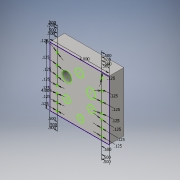
# Autodesk Inventor part: PopQuiz
Saved by Autodesk Inventor 2016 (Build 200138000, 138)
## iProperties
Created: 2018-02-16
Part Number: PopQuiz
Material: Generic
Document SubType Name: Modeling
Designer: sun01147
Density: 1 g/cm^3
Appearance: Default
Author: sun01147
Autodesk Inventor part; units mm, degrees
ref_plane "YZ Plane" through (0, 0, 0) normal (1, 0, 0) x (0, 1, 0)
ref_plane "XZ Plane" through (0, 0, 0) normal (0, 1, 0) x (-1, 0, 0)
ref_plane "XY Plane" through (0, 0, 0) normal (0, 0, 1) x (1, 0, 0)
sketch "Sketch1" plane through (0, 0, 0) normal (0, 0, 1) x (1, 0, 0)
  line L0 (0, 0) -> (0, 101.6)
  line L1 (0, 101.6) -> (101.6, 101.6)
  line L2 (101.6, 101.6) -> (101.6, 0)
  line L3 (101.6, 0) -> (0, 0)
  circle A0 centre (12.7, 92.4868) radius 1.5875
  circle A1 centre (12.7, 73.555) radius 1.5875
  circle A2 centre (12.7, 57.3937) radius 1.5875
  circle A3 centre (12.7, 43.772) radius 1.5875
  circle A4 centre (12.7, 31.3047) radius 1.5875
  circle A5 centre (12.7, 18.1448) radius 1.5875
  circle A6 centre (12.7, 5.9084) radius 1.5875
  circle A7 centre (88.9, 92.4868) radius 1.5875
  circle A8 centre (88.9, 73.555) radius 1.5875
  circle A9 centre (88.9, 57.3937) radius 1.5875
  circle A10 centre (88.9, 39.5628) radius 1.5875
  circle A11 centre (88.9, 31.3047) radius 1.5875
  circle A12 centre (88.9, 18.1448) radius 1.5875
  circle A13 centre (88.9, 5.9084) radius 1.5875
  circle A14 centre (50.8, 81.1516) radius 6.818
  circle A15 centre (29.171, 64.7351) radius 8.5087
  circle A16 centre (29.171, 31.3047) radius 5.8892
  circle A17 centre (52.7512, 14.59) radius 5.559
  circle A18 centre (70.9586, 37.1939) radius 6.2089
  circle A19 centre (70.9586, 60.8548) radius 7.7442
  dimension "d0" = 101.6
  dimension "d1" = 101.6
  dimension "d2" = 3.175
  dimension "d3" = 3.175
  dimension "d4" = 3.175
  dimension "d5" = 3.175
  dimension "d6" = 3.175
  dimension "d7" = 3.175
  dimension "d8" = 3.175
  dimension "d9" = 12.7
  dimension "d10" = 12.7
  dimension "d11" = 12.7
  dimension "d12" = 12.7
  dimension "d13" = 12.7
  dimension "d14" = 12.7
  dimension "d15" = 12.7
  dimension "d18" = 3.175
  dimension "d19" = 3.175
  dimension "d20" = 3.175
  dimension "d21" = 3.175
  dimension "d22" = 3.175
  dimension "d23" = 3.175
  dimension "d24" = 3.175
  dimension "d25" = 12.7
  dimension "d26" = 12.7
  dimension "d27" = 12.7
  dimension "d28" = 12.7
  dimension "d29" = 12.7
  dimension "d30" = 12.7
  dimension "d31" = 12.7
  constraints: 20 centre point, 8 end point, 2 perpendicular, 2 vertical
  measures "d0" distance of L0.start L0.end
  measures "d1" distance of L0.end L1.end
  measures "d2" diameter of A0
  measures "d3" diameter of A1
  measures "d4" diameter of A2
  measures "d5" diameter of A3
  measures "d6" diameter of A4
  measures "d7" diameter of A5
  measures "d8" diameter of A6
  measures "d9" distance from line of A0.centre L0
  measures "d10" distance from line of L0 A1.centre
  measures "d11" distance from line of L0 A2.centre
  measures "d12" distance from line of L0 A3.centre
  measures "d13" distance from line of L0 A4.centre
  measures "d14" distance from line of L0 A5.centre
  measures "d15" distance from line of L0 A6.centre
  measures "d18" diameter of A7
  measures "d19" diameter of A8
  measures "d20" diameter of A9
  measures "d21" diameter of A10
  measures "d22" diameter of A11
  measures "d23" diameter of A12
  measures "d24" diameter of A13
  measures "d25" distance from line of L2 A7.centre
  measures "d26" distance from line of L2 A8.centre
  measures "d27" distance from line of L2 A9.centre
  measures "d28" distance from line of L2 A10.centre
  measures "d29" distance from line of L2 A11.centre
  measures "d30" distance from line of L2 A12.centre
  measures "d31" distance from line of L2 A13.centre
extrude "Extrusion1" add sketch "Sketch1" against normal blind 25.4 contours L0 L1 L2 L3 | A7 | A8 | A9 | A10 | A11 | A12 | A13 | A14 | A15 | A16 | A17 | A18 | A19
extrude "Extrusion2" cut sketch "Sketch1" against normal blind 25.4 contours A7
extrude "Extrusion3" cut sketch "Sketch1" against normal blind 25.4 contours A8
extrude "Extrusion4" cut sketch "Sketch1" against normal blind 25.4 contours A9
extrude "Extrusion5" cut sketch "Sketch1" against normal blind 25.4 contours A10
extrude "Extrusion6" cut sketch "Sketch1" against normal blind 25.4 contours A11
extrude "Extrusion7" cut sketch "Sketch1" against normal blind 25.4 contours A12
extrude "Extrusion8" cut sketch "Sketch1" against normal blind 25.4 contours A13
extrude "Extrusion9" cut sketch "Sketch1" against normal blind 25.4 contours A15
body "Solid1"
